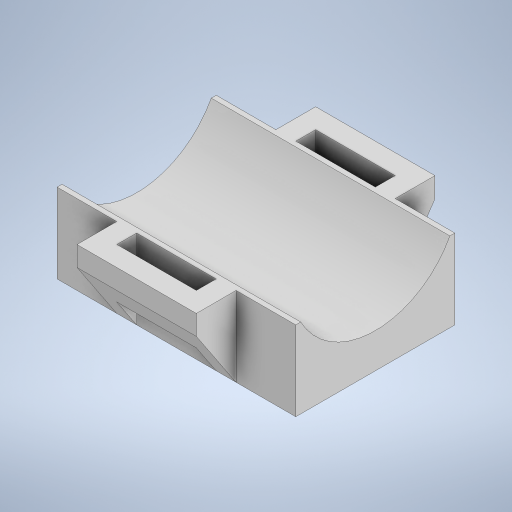
# Autodesk Inventor part: Part_4_scooter_attachment
Saved by Autodesk Inventor 2023 (Build 270158000, 158)
## iProperties
Created: 2023-09-30
Part Number: Part_4_scooter_attachment
Material: Generic
Document SubType Name: Modeling
Designer: zskus
Density: 1 g/cm^3
Appearance: Default
Author: zskus
Autodesk Inventor part; units mm, degrees
ref_plane "YZ Plane" through (0, 0, 0) normal (1, 0, 0) x (0, 1, 0)
ref_plane "XZ Plane" through (0, 0, 0) normal (0, 1, 0) x (-1, 0, 0)
ref_plane "XY Plane" through (0, 0, 0) normal (0, 0, 1) x (1, 0, 0)
sketch "Sketch1" plane through (0, 0, 0) normal (0, 1, 0) x (-1, 0, 0)
  line L0 (-38.1, 25.4) -> (38.1, 25.4)
  line L1 (38.1, 25.4) -> (38.1, -25.4)
  line L2 (38.1, -25.4) -> (-38.1, -25.4)
  line L3 (-38.1, -25.4) -> (-38.1, 25.4)
  point P0 (0, 0)
  dimension "d0" = 50.8
  dimension "d1" = 76.2
  dimension "d2" = 25.4
  dimension "d3" = 38.1
  constraints: 8 end point, 2 parallel, 1 horizontal, 1 perpendicular
  measures "d0" distance of L0.end L1.end
  measures "d1" distance of L1.end L2.end
  measures "d2" distance from line of point (0, 0) L0
  measures "d3" distance from line of L3 point (0, 0)
extrude "Extrusion1" add sketch "Sketch1" along normal blind 25.4
sketch "Sketch2" plane through (38.1, 0, 25.4) normal (1, 0, 0) x (0, 0, -1)
  circle A0 centre (25.4, 38.1) radius 26.9875
  line L0 (0, 0) -> (50.8, 0) projected
  line L1 (50.8, 0) -> (50.8, 25.4) projected
  line L2 (0, 25.4) -> (50.8, 25.4) projected
  line L3 (0, 0) -> (0, 25.4) projected
  point P0 (25.4, 0)
  dimension "d6" = 53.975
  constraints: 1 centre point
  measures "d6" diameter of A0
extrude "Extrusion2" cut sketch "Sketch2" against normal through all contours A0 L2 | L2 A0
sketch "Sketch3" plane through (0, 0, 0) normal (0, -1, 0) x (1, 0, 0)
  line L0 (38.1, -25.4) -> (-38.1, -25.4) projected
  line L1 (19.05, -25.4) -> (-19.05, -25.4)
  line L2 (-19.05, -25.4) -> (-19.05, -38.1)
  line L3 (19.05, -38.1) -> (19.05, -25.4)
  line L4 (12.7, -25.4) -> (-12.7, -25.4)
  line L5 (-12.7, -25.4) -> (-12.7, -31.75)
  line L6 (-12.7, -31.75) -> (12.7, -31.75)
  line L7 (12.7, -31.75) -> (12.7, -25.4)
  line L8 (38.1, -25.4) -> (-38.1, -25.4) projected
  line L9 (38.1, 25.4) -> (38.1, -25.4) projected
  line L10 (-38.1, 25.4) -> (38.1, 25.4) projected
  line L11 (-38.1, -25.4) -> (-38.1, 25.4) projected
  line L12 (-19.05, -38.1) -> (19.05, -38.1)
  point P0 (0, 0)
  point P1 (12.7, -28.575)
  dimension "d10" = 25.4
  dimension "d11" = 6.35
  dimension "d12" = 6.35
  dimension "d13" = 6.35
  dimension "d14" = 6.35
  dimension "d16" = 12.7
  constraints: 16 end point, 3 horizontal, 3 parallel, 2 perpendicular, 2 point on line, 1 midpoint
  measures "d10" distance of L5.end L6.end
  measures "d11" distance from line of L3 point (12.7, -28.575)
  measures "d12" distance between parallel lines of L5 L2
  measures "d13" distance between parallel lines of L6 L12
  measures "d14" distance between parallel lines of L4 L6
  measures "d16" distance from line of point (0, 0) L7
extrude "Extrusion3" add sketch "Sketch3" against normal blind 25.4 contours L3 L12 L2 L0 L5 L6 L7
sketch "Sketch4" plane through (19.05, 0, -25.4) normal (1, 0, 0) x (0, 0, -1)
  line L0 (12.7, 0) -> (0, 0) projected
  line L1 (12.7, 0) -> (12.7, 25.4) projected
  line L2 (0, 25.4) -> (12.7, 25.4) projected
  line L3 (0, 0) -> (0, 25.4) projected
  arc A0 (-49.2125, 25.4) -> (-1.5875, 25.4) centre (-25.4, 38.1) ccw projected
  line L4 (-50.8, 25.4) -> (-49.2125, 25.4) projected
  line L5 (-50.8, 0) -> (-50.8, 25.4) projected
  line L6 (-50.8, 0) -> (0, 0) projected
  line L7 (0, 0) -> (0, 25.4) projected
  line L8 (-1.5875, 25.4) -> (0, 25.4) projected
  line L9 (6.35, 0) -> (0, 0) projected
  line L10 (0, 0) -> (12.7, 19.05)
  line L11 (12.7, 0) -> (12.7, 25.4) projected
  point P0 (-25.4, 0)
  point P1 (12.7, 19.05)
  dimension "d19" = 6.35
  constraints: 2 end point, 1 point on line
  measures "d19" distance from line of L2 L10.end
extrude "Extrusion4" cut sketch "Sketch4" against normal through all contours L0 L10 L1
mirror "Mirror1" about plane through (0, 0, 0) normal (0, 0, 1) of "Extrusion3", "Extrusion4"
equation "\"d2\" = 0.5 * d0"
equation "\"d3\" = 0.5 * d1"
equation "\"d12\" = d11"
equation "\"d13\" = d11"
equation "\"d16\" = 0.5 * d10"
body "Solid1"
